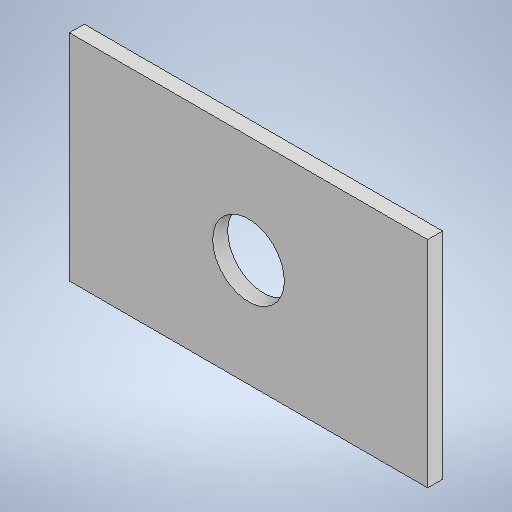
# Autodesk Inventor part: rectangle
Saved by Autodesk Inventor 2025.1 (Build 291241000, 241)
## iProperties
Created: 2024-11-06
Part Number: rectangle
Material: Generic
Document SubType Name: Modeling
Designer: bless
Density: 1 g/cm^3
Appearance: Default
Author: bless
Autodesk Inventor part; units mm, degrees
ref_plane "YZ Plane" through (0, 0, 0) normal (1, 0, 0) x (0, 1, 0)
ref_plane "XZ Plane" through (0, 0, 0) normal (0, 1, 0) x (-1, 0, 0)
ref_plane "XY Plane" through (0, 0, 0) normal (0, 0, 1) x (1, 0, 0)
sketch "Sketch1" plane through (0, 0, 0) normal (0, 0, 1) x (1, 0, 0)
  line L0 (-76.2, 45.72) -> (76.2, 45.72)
  line L1 (76.2, 45.72) -> (76.2, -45.72)
  line L2 (76.2, -45.72) -> (-76.2, -45.72)
  line L3 (-76.2, -45.72) -> (-76.2, 45.72)
  circle A0 centre (0, 0) radius 15.24
  dimension "d0" = 152.4
  dimension "d1" = 91.44
  dimension "d2" = 76.2
  dimension "d3" = 45.72
  dimension "d4" = 30.48
  constraints: 8 end point, 2 parallel, 1 centre point, 1 coincident, 1 horizontal, 1 perpendicular
  measures "d0" distance of L0.start L0.end
  measures "d1" distance of L2.end L0.start
  measures "d2" horizontal distance of L1.end point (0, 0)
  measures "d3" distance from line of point (0, 0) L0
  measures "d4" diameter of A0
extrude "Extrusion1" add sketch "Sketch1" along normal blind 6.35
equation "\"d2\" = 0.5 * d0"
equation "\"d3\" = 0.5 * d1"
equation "\"d4\" = 0.333333 * d1"
body "Solid1"
